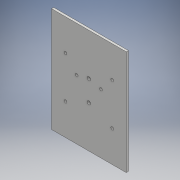
# Autodesk Inventor part: base superior
Saved by Autodesk Inventor 2018 (Build 220112000, 112)
## iProperties
Created: 2019-05-16
Part Number: base superior
Material: Generic
Document SubType Name: Modeling
Designer: JLVega003
Density: 1 g/cm^3
Appearance: Default
Author: JLVega003
Autodesk Inventor part; units mm, degrees
ref_plane "YZ Plane" through (0, 0, 0) normal (1, 0, 0) x (0, 1, 0)
ref_plane "XZ Plane" through (0, 0, 0) normal (0, 1, 0) x (-1, 0, 0)
ref_plane "XY Plane" through (0, 0, 0) normal (0, 0, 1) x (1, 0, 0)
sketch "Sketch1" plane through (0, 0, 0) normal (0, 1, 0) x (-1, 0, 0)
  line L0 (53.5, 75) -> (-53.5, 75)
  line L1 (-53.5, 75) -> (-53.5, -75)
  line L2 (-53.5, -75) -> (53.5, -75)
  line L3 (53.5, -75) -> (53.5, 75)
  line L4 (74.9, 0) -> (-74.9, 0) projected
  line L5 (0, -105) -> (0, 105) projected
  point P0 (0, 0)
  point P1 (0, 75)
  point P2 (53.5, 0)
  dimension "d0" = 150
  dimension "d1" = 107
  constraints: 8 end point, 2 midpoint, 2 parallel, 2 point on line, 1 horizontal, 1 perpendicular
  measures "d0" distance between parallel lines of L2 L0
  measures "d1" distance between parallel lines of L1 L3
extrude "Extrusion1" add sketch "Sketch1" along normal blind 3.175
sketch "Sketch2" plane through (0, 3.175, 0) normal (0, 1, 0) x (1, 0, 0)
  line L0 (-53.5, -75) -> (53.5, -75) projected
  line L1 (-53.5, 75) -> (-53.5, -75) projected
  line L2 (53.5, 75) -> (-53.5, 75) projected
  line L3 (-33.5, -30) -> (33.5, -30)
  line L4 (33.5, -30) -> (33.5, 30) construction
  line L5 (33.5, 30) -> (-33.5, 30) construction
  line L6 (-33.5, 30) -> (-33.5, -30) construction
  line L7 (-74.9, 0) -> (74.9, 0) projected
  line L8 (0, 105) -> (0, -105) projected
  line L9 (-17.5, -10.5) -> (17.5, -10.5)
  point P0 (0, -30)
  point P1 (-33.5, 0)
  point P2 (0, -10.5)
  point P3 (0, -15)
  point P4 (0, 15)
  dimension "d11" = 45
  dimension "d12" = 20
  dimension "d13" = 64.5
  dimension "d14" = 35
  dimension "d15" = 15
  dimension "d16" = 15
  constraints: 10 end point, 5 point on line, 4 coincident, 3 midpoint, 3 parallel, 1 horizontal, 1 perpendicular
  measures "d11" distance between parallel lines of L3 L0
  measures "d12" distance between parallel lines of L1 L6
  measures "d13" distance between parallel lines of L9 L0
  measures "d14" distance of L9.start L9.end
  measures "d15" distance from line of L7 point (0, -15)
  measures "d16" distance from line of point (0, 15) L7
hole "Hole1" at (-17.5, 3.175, 10.5) at (17.5, 3.175, 10.5) at (-33.5, 3.175, 30) at (-33.5, 3.175, -30) at (33.5, 3.175, -30) at (33.5, 3.175, 30) direction (0, -1, 0) diameter 4 end through all
hole "Hole2" at (0, 3.175, 15) at (0, 3.175, -15) direction (0, -1, 0) diameter 5 end through all
equation "\"d16\" = d15"
body "Solid1"
